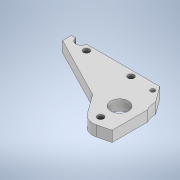
# Autodesk Inventor part: Claw_Finger
Saved by Autodesk Inventor 2022 (Build 260153000, 153)
## iProperties
Created: 2022-03-18
Part Number: Claw_Finger
Material: Generic
Document SubType Name: Modeling
Designer: Mlees
Density: 1 g/cm^3
Appearance: Default
Author: Mlees
Autodesk Inventor part; units mm, degrees
ref_plane "YZ Plane" through (0, 0, 0) normal (1, 0, 0) x (0, 1, 0)
ref_plane "XZ Plane" through (0, 0, 0) normal (0, 1, 0) x (-1, 0, 0)
ref_plane "XY Plane" through (0, 0, 0) normal (0, 0, 1) x (1, 0, 0)
sketch "Sketch1" plane through (0, 0, 0) normal (0, 1, 0) x (-1, 0, 0)
  line L0 (8, -38) -> (1.5, -29.1259)
  arc A0 (1.5, -29.1259) -> (0, -23) centre (-10.496, -28.8167) ccw
  line L1 (0, -23) -> (0, -3)
  line L2 (0, -3) -> (12.1347, 0)
  line L3 (58, -38) -> (58, -33)
  line L4 (23, -15) -> (58, -33)
  line L5 (23, -15) -> (12.1347, 0)
  circle A1 centre (9.75, -6.25) radius 1.75
  line L6 (0, 0) -> (0, -17)
  circle A2 centre (9.75, -17) radius 5
  circle A3 centre (8, -34) radius 1.25
  circle A4 centre (46.25, -34.75) radius 1.75
  circle A5 centre (21, -34.75) radius 1.75
  line L7 (58, -38) -> (55.5, -38)
  arc A6 (55.5, -38) -> (49.5, -38) centre (52.5, -38) ccw
  line L8 (58, -38) -> (55.5, -38)
  line L9 (49.5, -38) -> (8, -38)
  dimension "d2" = 50
  dimension "d6" = 11
  dimension "d7" = 12
  dimension "d8" = 20
  dimension "d15" = 3.5
  dimension "d16" = 17
  dimension "d17" = 10
  dimension "d23" = 2.5
  dimension "d26" = 3.5
  dimension "d28" = 2.5
  dimension "d30" = 3
  constraints: 20 end point, 7 centre point, 4 point on circle, 1 point on line
  measures "d2" distance of L3.start L0.start
  measures "d6" distance of L0.end L0.start
  measures "d7" radius of A0
  measures "d8" distance of L1.start L1.end
  measures "d15" diameter of A1
  measures "d16" distance of L6.start L6.end
  measures "d17" diameter of A2
  measures "d23" diameter of A3
  measures "d26" diameter of A4
  measures "d28" distance of L3.start L7.end
  measures "d30" radius of A6
extrude "Extrusion1" add sketch "Sketch1" along normal blind 6
fillet "Fillet1" radius 7.5 1 edges at (-12.1347, 3, 0)
body "Solid1"
